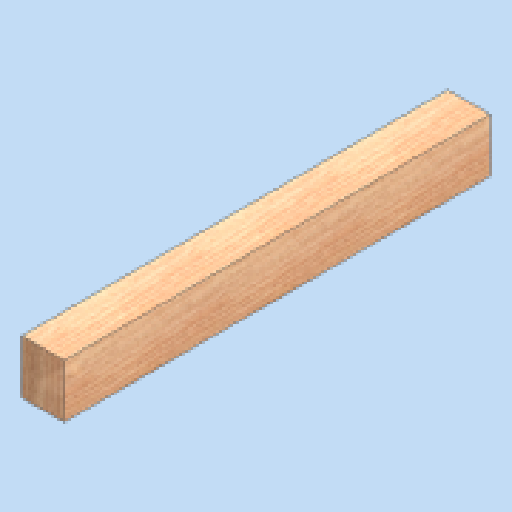
# Autodesk Inventor part: PoutreDirection
Saved by Autodesk Inventor 2023 (Build 270158000, 158)
## iProperties
Created: 2026-03-22
Part Number: PoutreDirection
Material: Wood (Birch)
Document SubType Name: Modeling
Designer: Nathann
Density: 0.55 g/cm^3
Appearance: Birch - Natural Polished
Author: Nathann
Autodesk Inventor part; units mm, degrees
ref_plane "YZ Plane" through (0, 0, 0) normal (1, 0, 0) x (0, 1, 0)
ref_plane "XZ Plane" through (0, 0, 0) normal (0, 1, 0) x (-1, 0, 0)
ref_plane "XY Plane" through (0, 0, 0) normal (0, 0, 1) x (1, 0, 0)
sketch "Sketch1" plane through (0, 0, 0) normal (0, 0, 1) x (1, 0, 0)
  line L0 (0, 0) -> (-80, 0)
  line L1 (-80, 0) -> (-80, 100)
  line L2 (-80, 100) -> (0, 100)
  line L3 (0, 100) -> (0, 0)
  dimension "d0" = 100
  dimension "d1" = 80
  constraints: 8 end point, 2 parallel, 1 horizontal, 1 perpendicular
  measures "d0" distance of L2.end L0.start
  measures "d1" distance of L1.end L2.end
extrude "Extrusion1" add sketch "Sketch1" along normal blind 800
body "Solid1"
